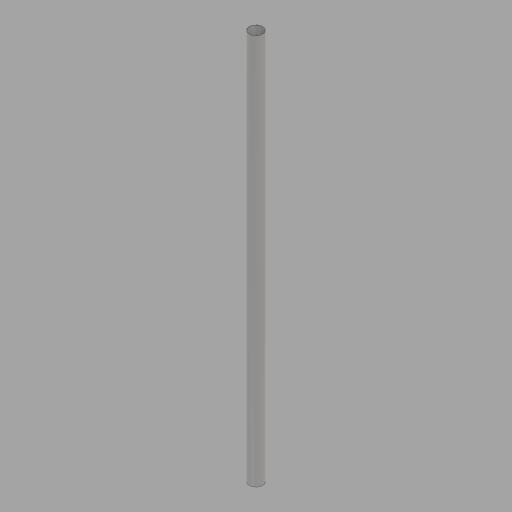
# Autodesk Inventor part: cylinder
Saved by Autodesk Inventor 2024 (Build 280153020, 153B)
## iProperties
Created: 2023-10-26
Part Number: cylinder
Material: Stainless Steel
Document SubType Name: Modeling
Designer: schanen
Density: 8 g/cm^3
Appearance: Semi-Polished
Mass: 2240.03 g
Surface Area: 3504.36 cm^2
Volume: 280.004 cm^3
cylinder_od: 44.450 mm
cylinder_wall: 0.380 mm
Author: schanen
Autodesk Inventor part; units mm, degrees
ref_plane "YZ Plane" through (0, 0, 0) normal (1, 0, 0) x (0, 1, 0)
ref_plane "XZ Plane" through (0, 0, 0) normal (0, 1, 0) x (-1, 0, 0)
ref_plane "XY Plane" through (0, 0, 0) normal (0, 0, 1) x (1, 0, 0)
sketch "Sketch1" plane through (0, 0, 0) normal (0, 1, 0) x (-1, 0, 0)
  circle A0 centre (0, 0) radius 22.225
  circle A1 centre (0, 0) radius 21.845
  dimension "cylinder_od" = 44.45
  dimension "cylinder_wall" = 0.38
  constraints: 2 centre point, 2 coincident
  measures "cylinder_od" diameter of A0
  measures "cylinder_wall" radial gap between concentric circles of A0 A1
extrude "Extrusion1" add sketch "Sketch1" along normal blind 1300
body "Solid1"
